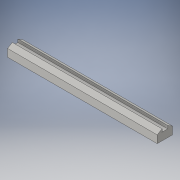
# Autodesk Inventor part: Bed Rail Connecting Pin
Saved by Autodesk Inventor 2016 (Build 200138000, 138)
## iProperties
Created: 2016-03-27
Part Number: Bed Rail Connecting Pin
Material: Generic
Document SubType Name: Modeling
Designer: Scott
Density: 1 g/cm^3
Appearance: Default
Author: Scott
Autodesk Inventor part; units mm, degrees
ref_plane "YZ Plane" through (0, 0, 0) normal (1, 0, 0) x (0, 1, 0)
ref_plane "XZ Plane" through (0, 0, 0) normal (0, 1, 0) x (-1, 0, 0)
ref_plane "XY Plane" through (0, 0, 0) normal (0, 0, 1) x (1, 0, 0)
sketch "Sketch1" plane through (0, 0, 0) normal (1, 0, 0) x (0, 1, 0)
  line L0 (-2.54, 5.08) -> (2.54, 5.08)
  line L1 (2.54, 5.08) -> (2.54, -5.08)
  line L2 (2.54, -5.08) -> (-2.54, -5.08)
  line L3 (-2.54, -5.08) -> (-2.54, 5.08)
  line L4 (-2.54, 5.08) -> (2.54, -5.08) construction
  line L5 (2.54, 5.08) -> (-2.54, -5.08) construction
  line L6 (2.54, 0) -> (2.54, -1.905)
  line L7 (2.54, -1.905) -> (4.445, -1.905)
  line L8 (4.445, -1.905) -> (2.54, -5.08)
  line L9 (2.54, 0) -> (2.54, 1.905)
  line L10 (2.54, 1.905) -> (4.445, 1.905)
  line L11 (4.445, 1.905) -> (2.54, 5.08)
  point P0 (0, 0)
  dimension "d0" = 5.08
  dimension "d1" = 10.16
  dimension "d2" = 1.905
  dimension "d3" = 1.905
  dimension "d4" = 1.905
  constraints: 24 end point, 3 midpoint, 3 perpendicular, 2 parallel, 2 point on line, 1 horizontal
  measures "d0" distance of L1.end L2.end
  measures "d1" distance of L0.end L1.end
  measures "d2" distance of L6.start L6.end
  measures "d3" distance of L6.end L7.end
  measures "d4" distance of L6.start L9.end
extrude "Extrusion1" add sketch "Sketch1" along normal blind 100
body "Solid1"
